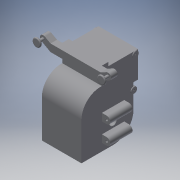
# Autodesk Inventor part: Front_Diff
Saved by Autodesk Inventor 2019 (Build 230136000, 136)
## iProperties
Created: 2019-03-02
Part Number: Front_Diff
Material: Generic
Document SubType Name: Modeling
Designer: alarr
Density: 1 g/cm^3
Appearance: Default
Author: alarr
Autodesk Inventor part; units mm, degrees
ref_plane "YZ Plane" through (0, 0, 0) normal (1, 0, 0) x (0, 1, 0)
ref_plane "XZ Plane" through (0, 0, 0) normal (0, 1, 0) x (-1, 0, 0)
ref_plane "XY Plane" through (0, 0, 0) normal (0, 0, 1) x (1, 0, 0)
sketch "Sketch2" plane through (0, 0, 0) normal (1, 0, 0) x (0, 1, 0)
  arc A0 (-27.94, 0) -> (0, -27.94) centre (0, 0) ccw
  arc A1 (-0.3456, 27.9379) -> (49.53, 15.24) centre (23.4285, 17.018) ccw construction
  line L0 (0, -27.94) -> (68.58, -27.94)
  line L1 (68.58, -27.94) -> (68.58, 15.24)
  line L2 (68.58, 15.24) -> (49.53, 15.24)
  line L3 (0, 0) -> (-27.94, 0) construction
  line L4 (23.4285, 43.18) -> (-27.94, 43.18)
  line L5 (-27.94, 43.18) -> (-27.94, 0)
  arc A2 (23.4285, 43.18) -> (-0.3456, 27.9379) centre (23.4285, 17.018) ccw construction
  arc A3 (49.53, 15.24) -> (23.4285, 43.18) centre (23.4285, 17.018) ccw
  arc A4 (-0.3456, 27.9379) -> (-27.94, 0) centre (0, 0) ccw construction
  arc A5 (0, -27.94) -> (-0.3456, 27.9379) centre (0, 0) ccw construction
  dimension "d0" = 55.88
  dimension "d1" = 52.324
  dimension "d2" = 43.18
  dimension "d3" = 96.52
  dimension "d4" = 71.12
  dimension "d5" = 19.05
  constraints: 14 point on circle, 12 end point, 6 centre point, 6 tangent, 3 horizontal, 3 perpendicular, 1 coincident
  measures "d0" diameter of A0
  measures "d1" diameter of A1
  measures "d2" distance of L0.end L1.end
  measures "d3" distance from line of L1 L3.end
  measures "d4" distance between parallel lines of L4 L0
  measures "d5" distance of L1.end L2.end
extrude "Extrusion1" add sketch "Sketch2" along normal mid plane 54.102
sketch "Sketch3" plane through (-27.051, 49.53, 15.24) normal (0, 0, 1) x (1, 0, 0)
  line L0 (-7.239, 24.13) -> (61.341, 24.13)
  line L1 (61.341, 24.13) -> (61.341, 13.97) construction
  line L2 (61.341, 13.97) -> (-7.239, 13.97)
  line L3 (-7.239, 13.97) -> (-7.239, 24.13) construction
  line L4 (-7.239, 24.13) -> (61.341, 13.97) construction
  line L5 (61.341, 24.13) -> (-7.239, 13.97) construction
  line L6 (0, -77.47) -> (54.102, -77.47) projected
  line L7 (27.051, -77.47) -> (27.051, 24.13) construction
  line L8 (0, 19.05) -> (54.102, 19.05) projected
  line L9 (-7.239, 24.13) -> (-15.0178, 28.4339)
  line L10 (27.051, 256.9722) -> (27.051, 24.13) construction
  arc A0 (-15.0178, 28.4339) -> (-19.3216, 20.6551) centre (-17.1697, 24.5445) ccw
  line L11 (-19.3216, 20.6551) -> (-7.239, 13.97)
  arc A1 (-19.3216, 20.6551) -> (-15.0178, 28.4339) centre (-17.1697, 24.5445) ccw construction
  line L12 (61.341, 24.13) -> (69.1198, 28.4339)
  arc A2 (73.4236, 20.6551) -> (69.1198, 28.4339) centre (71.2717, 24.5445) ccw
  line L13 (73.4236, 20.6551) -> (61.341, 13.97)
  arc A3 (69.1198, 28.4339) -> (73.4236, 20.6551) centre (71.2717, 24.5445) ccw construction
  point P0 (27.051, -49.53)
  point P1 (27.051, 19.05)
  dimension "d8" = 10.16
  dimension "d9" = 68.58
  dimension "d10" = 5.08
  dimension "d17" = 8.89
  dimension "d19" = 8.89
  constraints: 24 end point, 8 point on circle, 4 centre point, 3 midpoint, 3 parallel, 3 symmetric about line, 2 tangent, 2 vertical, 1 horizontal, 1 perpendicular, 1 point on line, 2 other
  measures "d8" distance between parallel lines of L0 L2
  measures "d9" distance of L0.start L0.end
  measures "d10" distance between parallel lines of L8 L0
  measures "d17" distance of L0.start L9.end
  measures "d19" diameter of A0
extrude "Extrusion2" add sketch "Sketch3" along normal blind 8.89
sketch "Sketch4" plane through (-27.051, 49.53, 15.24) normal (0, 0, -1) x (-1, 0, 0)
  line L0 (7.239, 24.13) -> (-61.341, 24.13) projected
  line L1 (0, 19.05) -> (-54.102, 19.05) projected
  line L2 (-54.102, 13.97) -> (0, 13.97) projected
  line L3 (-61.341, 24.13) -> (7.239, 24.13) projected
  line L4 (-54.102, 13.97) -> (0, 13.97)
  line L5 (0, 13.97) -> (0, 24.13)
  line L6 (0, 24.13) -> (-54.102, 24.13)
  line L7 (-54.102, 24.13) -> (-54.102, 13.97)
  point P0 (-27.051, -49.53)
  constraints: 8 end point, 2 parallel, 1 horizontal, 1 perpendicular, 1 point on line
extrude "Extrusion3" add sketch "Sketch4" along normal blind 8.89
sketch "Sketch6" plane through (-27.051, 49.53, 24.13) normal (0, 0, 1) x (1, 0, 0)
  arc A0 (73.4236, 20.6551) -> (69.1198, 28.4339) centre (71.2717, 24.5445) ccw projected
  arc A1 (-15.0178, 28.4339) -> (-19.3216, 20.6551) centre (-17.1697, 24.5445) ccw projected
  circle A2 centre (-17.1697, 24.5445) radius 1.905
  circle A3 centre (71.2717, 24.5445) radius 1.905
  point P0 (27.051, -49.53)
  dimension "d20" = 3.81
  constraints: 2 centre point, 2 coincident, 1 equal radius
  measures "d20" diameter of A3
extrude "Extrusion4" cut sketch "Sketch6" against normal through all
sketch "Sketch7" plane through (27.051, 0, 0) normal (1, 0, 0) x (0, 0, -1)
  circle A0 centre (0, 0) radius 5.08
  dimension "d23" = 10.16
  constraints: 1 centre point, 1 coincident
  measures "d23" diameter of A0
extrude "Extrusion5" cut sketch "Sketch7" against normal blind 10.16
sketch "Sketch12" plane through (0, 0, 0) normal (1, 0, 0) x (0, 1, 0)
  line L0 (0, -27.94) -> (68.58, -27.94) projected
  line L1 (68.58, -27.94) -> (68.58, 6.35) projected
  line L2 (68.58, -27.94) -> (32.512, -27.94)
  line L3 (32.512, -27.94) -> (32.512, -34.29)
  line L4 (32.512, -34.29) -> (68.58, -34.29)
  line L5 (68.58, -34.29) -> (68.58, -27.94)
  point P0 (0, 0)
  dimension "d35" = 6.35
  dimension "d36" = 36.068
  constraints: 8 end point, 2 parallel, 1 horizontal, 1 perpendicular
  measures "d35" distance of L4.end L0.end
  measures "d36" distance of L3.end L4.end
extrude "Extrusion9" add sketch "Sketch12" along normal up to surface (54.102 mm away) from surface at -27.051
sketch "Sketch11" plane through (0, 0, 0) normal (1, 0, 0) x (0, 1, 0)
  circle A0 centre (23.4285, -27.94) radius 4.064
  line L0 (0, -27.94) -> (68.58, -27.94) projected
  arc A1 (49.53, 15.24) -> (23.4285, 43.18) centre (23.4285, 17.018) ccw construction
  circle A2 centre (23.4285, 17.018) radius 26.162 construction
  line L1 (23.4285, 17.018) -> (23.4285, -27.94) construction
  circle A3 centre (64.516, -30.226) radius 4.064
  line L2 (68.58, 6.35) -> (68.58, -34.29) projected
  line L3 (68.58, -34.29) -> (32.512, -34.29) projected
  point P0 (0, 0)
  dimension "d34" = 8.128
  constraints: 3 centre point, 2 end point, 2 equal radius, 2 tangent, 1 concentric, 1 point on line, 1 vertical
  measures "d34" diameter of A0
extrude "Extrusion10" add sketch "Sketch11" along normal mid plane 55.88 contours L0 A0 | A0 L0 | A3 L0 | L0 A3
sketch "Sketch13" plane through (27.94, 64.516, -30.226) normal (1, 0, 0) x (0, 0, -1)
  circle A0 centre (0, 0) radius 4.064 projected
  circle A1 centre (-2.286, -41.0875) radius 4.064 projected
  point P0 (-30.226, -64.516)
hole "Hole1" at (27.94, 64.516, -30.226) at (27.94, 23.4285, -27.94) direction (-1, 0, 0) diameter 1.9304 depth 25.4 tip angle 118
sketch "Sketch8" plane through (0, 0, 0) normal (0, 0, 1) x (1, 0, 0)
  arc A0 (28.321, 12.7) -> (33.401, 7.62) centre (33.401, 12.7) ccw construction
  line L0 (27.051, 23.4285) -> (27.051, -27.94) projected
  line L1 (33.401, 12.7) -> (27.051, 12.7) construction
  line L2 (33.401, 12.7) -> (33.401, 0) construction
  line L3 (0, 0) -> (33.401, 0) construction
  line L4 (33.401, 17.78) -> (27.051, 17.78)
  line L5 (33.401, 7.62) -> (27.051, 7.62)
  arc A1 (33.401, 17.78) -> (28.321, 12.7) centre (33.401, 12.7) ccw construction
  arc A2 (33.401, 7.62) -> (33.401, 17.78) centre (33.401, 12.7) ccw
  point P0 (27.051, 0)
  dimension "d26" = 10.16
  dimension "d27" = 6.35
  dimension "d28" = 12.7
  constraints: 10 end point, 6 point on circle, 4 point on line, 4 tangent, 3 centre point, 3 perpendicular, 1 horizontal, 1 vertical
  measures "d26" diameter of A0
  measures "d27" distance of L1.start L1.end
  measures "d28" distance of L1.start L2.end
extrude "Extrusion6" add sketch "Sketch8" along normal mid plane 30.48
sketch "Sketch9" plane through (0, 0, 15.24) normal (0, 0, 1) x (1, 0, 0)
  arc A0 (33.401, 7.62) -> (33.401, 17.78) centre (33.401, 12.7) ccw projected
  circle A1 centre (33.401, 12.7) radius 1.5875
  point P0 (0, 0)
  dimension "d31" = 3.175
  constraints: 1 centre point, 1 coincident
  measures "d31" diameter of A1
extrude "Extrusion7" cut sketch "Sketch9" against normal through all
mirror "Mirror1" about plane through (0, 0, 0) normal (0, 1, 0) of "Extrusion6", "Extrusion7"
sketch "Sketch15" plane through (-27.051, 49.53, 24.13) normal (0, 0, 1) x (1, 0, 0)
  circle A0 centre (71.2717, 24.5445) radius 1.905 projected
  circle A1 centre (71.2717, 24.5445) radius 1.905
  point P0 (27.051, -49.53)
  constraints: 1 centre point, 1 coincident, 1 concentric
extrude "Extrusion11" add sketch "Sketch15" along normal mid plane 13.97
sketch "Sketch16" plane through (44.2207, 74.0745, 31.115) normal (0, 0, 1) x (1, 0, 0)
  circle A0 centre (0, 0) radius 1.905 projected
  circle A1 centre (0, 0) radius 5.715
  point P0 (-44.2207, -74.0745)
  dimension "d52" = 3.81
  constraints: 1 centre point
  measures "d52" radial gap between concentric circles of A0 A1
extrude "Extrusion12" add sketch "Sketch16" along normal blind 2.54 contours A0 | A1
full round fillet "Fillet1" first side at (48.5919, 73.4666, 31.115) centre faces at (49.9171, 73.6146, 32.8083) second side at (43.1214, 74.0124, 33.655)
mirror "Mirror2" about plane through (0, 0, 0) normal (1, 0, 0) of "Extrusion6", "Extrusion7", "Mirror1", "Hole1", "Extrusion5", "Extrusion11", "Extrusion12", "Fillet1"
body "Solid1"
